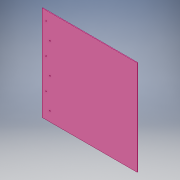
# Autodesk Inventor part: Door
Saved by Autodesk Inventor 2018 (Build 220112000, 112)
## iProperties
Created: 2018-10-16
Part Number: Door
Material: Steel
Document SubType Name: Modeling
Designer: P301319
Density: 7.85 g/cm^3
Appearance: Pink
Author: P301319
Autodesk Inventor part; units mm, degrees
ref_plane "YZ Plane" through (0, 0, 0) normal (1, 0, 0) x (0, 1, 0)
ref_plane "XZ Plane" through (0, 0, 0) normal (0, 1, 0) x (-1, 0, 0)
ref_plane "XY Plane" through (0, 0, 0) normal (0, 0, 1) x (1, 0, 0)
sketch "Sketch1" plane through (0, 0, 0) normal (0, 1, 0) x (-1, 0, 0)
  line L0 (0, 0) -> (-250, 0)
  line L1 (-250, 0) -> (-250, -250)
  line L2 (-250, -250) -> (0, -250)
  line L3 (0, -250) -> (0, 0)
  dimension "d0" = 250
  dimension "d1" = 250
  constraints: 8 end point, 2 parallel, 1 horizontal, 1 perpendicular
  measures "d0" distance of L2.end L1.end
  measures "d1" distance of L1.end L0.end
extrude "Extrusion1" add sketch "Sketch1" along normal blind 1.6
sketch "Sketch2" plane through (0, 0, 0) normal (0, -1, 0) x (1, 0, 0)
  line L0 (0, -250) -> (0, 0) projected
  line L1 (0, 0) -> (250, 0) projected
  point P0 (10, -25)
  point P1 (10, -105)
  point P2 (10, -185)
  point P3 (20, -225)
  point P4 (20, -145)
  point P5 (20, -65)
  dimension "d4" = 10
  dimension "d5" = 10
  dimension "d6" = 40
  dimension "d7" = 40
  dimension "d8" = 40
  dimension "d9" = 40
  dimension "d10" = 40
  dimension "d11" = 25
  constraints: 4 vertical alignment
  measures "d4" distance from line of L0 point (10, -25)
  measures "d5" horizontal distance of point (10, -25) point (20, -65)
  measures "d6" vertical distance of point (20, -65) point (10, -25)
  measures "d7" vertical distance of point (20, -65) point (10, -105)
  measures "d8" vertical distance of point (10, -105) point (20, -145)
  measures "d9" vertical distance of point (20, -145) point (10, -185)
  measures "d10" vertical distance of point (10, -185) point (20, -225)
  measures "d11" distance from line of L1 point (10, -25)
hole "Hole1" at (10, 0, -25) at (10, 0, -105) at (10, 0, -185) at (20, 0, -225) at (20, 0, -145) at (20, 0, -65) direction (0, 1, 0) diameter 3 end through all
equation "\"d7\" = d6"
equation "\"d8\" = d6"
equation "\"d9\" = d6"
equation "\"d10\" = d6"
body "Solid1"
